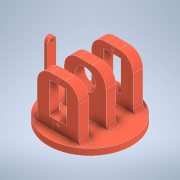
# Autodesk Inventor part: PIEZA 2
Saved by Autodesk Inventor 2021 (Build 250183000, 183)
## iProperties
Created: 2021-03-25
Part Number: PIEZA 2
Material: Generic
Document SubType Name: Modeling
Designer: LRC
Density: 1 g/cm^3
Appearance: Generic
Author: LRC
Autodesk Inventor part; units mm, degrees
ref_plane "YZ Plane" through (0, 0, 0) normal (1, 0, 0) x (0, 1, 0)
ref_plane "XZ Plane" through (0, 0, 0) normal (0, 1, 0) x (-1, 0, 0)
ref_plane "XY Plane" through (0, 0, 0) normal (0, 0, 1) x (1, 0, 0)
sketch "Sketch2" plane through (0, 0, 0) normal (0, 1, 0) x (-1, 0, 0)
  circle A0 centre (0, 0) radius 30
  dimension "d3" = 60
  constraints: 1 centre point, 1 coincident
  measures "d3" diameter of A0
extrude "Extrusion2" add sketch "Sketch2" along normal blind 4.5
sketch "Sketch3" plane through (0, 4.5, 0) normal (0, 1, 0) x (1, 0, 0)
  line L0 (-15, 0) -> (15, 0)
  line L1 (0, -3.5) -> (0, 3.5)
  line L2 (-15, 0) -> (-15, -3.5)
  line L3 (-15, -3.5) -> (15, -3.5)
  line L4 (15, -3.5) -> (15, 3.5)
  line L5 (15, 3.5) -> (-15, 3.5)
  line L6 (-15, 3.5) -> (-15, 0)
  line L7 (-15, -16) -> (-15, -23)
  line L8 (-15, -23) -> (15, -23)
  line L9 (15, -23) -> (15, -16)
  line L10 (15, -16) -> (-15, -16)
  line L11 (-15, 16) -> (-15, 23)
  line L12 (-15, 23) -> (15, 23)
  line L13 (15, 23) -> (15, 16)
  line L14 (15, 16) -> (-15, 16)
  point P0 (0, 0)
  point P1 (0, 0)
  point P2 (0, 0)
  dimension "d6" = 30
  dimension "d7" = 7
  dimension "d8" = 12.5
  dimension "d9" = 7
  dimension "d10" = 30
  dimension "d11" = 7
  constraints: 30 end point, 6 perpendicular, 4 symmetric about line, 3 coincident, 2 midpoint, 2 vertical, 1 horizontal, 1 point on line
  measures "d6" distance of L0.start L0.end
  measures "d7" distance of L1.start L1.end
  measures "d8" distance of L2.end L7.start
  measures "d9" distance of L7.start L7.end
  measures "d10" distance of L7.end L8.end
  measures "d11" distance of L8.end L9.end
extrude "Extrusion3" add sketch "Sketch3" along normal blind 35
fillet "Fillet1" radius 3 6 edges at (15, 4.5, 19.5) (15, 4.5, 0) (15, 4.5, -19.5) (-15, 4.5, 19.5) (-15, 4.5, 0) (-15, 4.5, -19.5)
fillet "Fillet2" radius 10 6 edges at (-15, 39.5, -19.5) (-15, 39.5, 0) (-15, 39.5, 19.5) (15, 39.5, -19.5) (15, 39.5, 0) (15, 39.5, 19.5)
sketch "Sketch4" plane through (0, 4.5, 0) normal (0, 1, 0) x (1, 0, 0)
  line L0 (0, 0) -> (0, 12.5)
  circle A0 centre (0, 12.5) radius 1.5
  line L1 (0, 0) -> (-7, 0)
  circle A1 centre (0, -12.5) radius 1.5
  dimension "d16" = 12.5
  dimension "d17" = 3
  constraints: 4 end point, 2 centre point, 1 coincident, 1 horizontal, 1 symmetric about line, 1 vertical, 1 other
  measures "d16" distance of L0.start L0.end
  measures "d17" diameter of A0
extrude "Extrusion4" cut sketch "Sketch4" against normal up to next
sketch "Sketch5" plane through (-18, 4.5, 23) normal (0, 0, 1) x (1, 0, 0)
  arc A0 (33, 25) -> (23, 35) centre (23, 25) ccw projected
  line L0 (13, 35) -> (23, 35) projected
  arc A1 (13, 35) -> (3, 25) centre (13, 25) ccw projected
  line L1 (3, 3) -> (3, 25) projected
  arc A2 (0, 0) -> (3, 3) centre (0, 3) ccw projected
  line L2 (36, 0) -> (0, 0) projected
  arc A3 (33, 3) -> (36, 0) centre (36, 3) ccw projected
  line L3 (33, 3) -> (33, 25) projected
  line L4 (3, 0) -> (18, 0)
  line L5 (18, 0) -> (18, 5)
  circle A4 centre (18, 5) radius 1
  line L6 (3, 35) -> (18, 35)
  line L7 (13, 35) -> (23, 35) projected
  line L8 (18, 30) -> (18, 35)
  line L9 (18, 35) -> (18, 32.5)
  circle A5 centre (18, 32.5) radius 1
  point P0 (18, -4.5)
  dimension "d20" = 15
  dimension "d21" = 5
  dimension "d22" = 2
  dimension "d23" = 15
  dimension "d24" = 5
  dimension "d25" = 2.5
  dimension "d26" = 2
  constraints: 10 end point, 3 midpoint, 2 centre point, 2 coincident, 1 perpendicular, 1 point on line
  measures "d20" distance of L4.start L4.end
  measures "d21" distance of L4.end L5.end
  measures "d22" diameter of A4
  measures "d23" distance of L6.start L6.end
  measures "d24" distance of L6.end L8.start
  measures "d25" distance of L6.end L9.end
  measures "d26" diameter of A5
extrude "Extrusion5" cut sketch "Sketch5" against normal blind 46 contours A4 | A5 L8 | L8 A5
sketch "Sketch6" plane through (-18, 4.5, 3.5) normal (0, 0, 1) x (1, 0, 0)
  circle A0 centre (18, 32.5) radius 1 projected
  circle A1 centre (18, 32.5) radius 1
  circle A2 centre (18, 5) radius 1
  point P0 (18, -4.5)
  constraints: 2 centre point, 1 coincident
extrude "Extrusion6" add sketch "Sketch6" against normal blind 7
sketch "Sketch7" plane through (-18, 4.5, 23) normal (0, 0, 1) x (1, 0, 0)
  circle A0 centre (18, 5) radius 1 projected
  circle A1 centre (18, 32.5) radius 1 projected
  arc A2 (33, 25) -> (23, 35) centre (23, 25) ccw projected
  line L0 (13, 35) -> (23, 35) projected
  arc A3 (13, 35) -> (3, 25) centre (13, 25) ccw projected
  line L1 (3, 3) -> (3, 25) projected
  arc A4 (0, 0) -> (3, 3) centre (0, 3) ccw projected
  line L2 (36, 0) -> (0, 0) projected
  arc A5 (33, 3) -> (36, 0) centre (36, 3) ccw projected
  line L3 (33, 3) -> (33, 25) projected
  line L4 (23, 35) -> (13, 35) projected
  line L5 (18, 35) -> (18, 30)
  line L6 (11.75, 30) -> (24.25, 30)
  line L7 (11.75, 30) -> (11.75, 7.5)
  line L8 (11.75, 7.5) -> (24.25, 7.5)
  line L9 (24.25, 7.5) -> (24.25, 30)
  point P0 (18, -4.5)
  dimension "d31" = 12.5
  dimension "d32" = 22.5
  constraints: 10 end point, 2 coincident, 2 midpoint, 2 perpendicular, 1 horizontal, 1 vertical
  measures "d31" distance of L6.start L6.end
  measures "d32" distance of L6.start L7.end
extrude "Extrusion7" cut sketch "Sketch7" against normal through all contours L6 L9 L8 L7
sketch "Sketch8" plane through (-18, 4.5, 3.5) normal (0, 0, 1) x (1, 0, 0)
  line L0 (13, 35) -> (23, 35) projected
  line L1 (18, 35) -> (18, 23.75)
  circle A0 centre (18, 23.75) radius 7.5
  line L2 (11.75, 7.5) -> (11.75, 30) projected
  line L3 (11.75, 30) -> (24.25, 30) projected
  line L4 (24.25, 30) -> (24.25, 7.5) projected
  line L5 (24.25, 7.5) -> (11.75, 7.5) projected
  arc A1 (33, 25) -> (23, 35) centre (23, 25) ccw projected
  line L6 (13, 35) -> (23, 35) projected
  arc A2 (13, 35) -> (3, 25) centre (13, 25) ccw projected
  line L7 (3, 3) -> (3, 25) projected
  arc A3 (0, 0) -> (3, 3) centre (0, 3) ccw projected
  line L8 (36, 0) -> (0, 0) projected
  arc A4 (33, 3) -> (36, 0) centre (36, 3) ccw projected
  line L9 (33, 3) -> (33, 25) projected
  line L10 (11.75, 30) -> (11.75, 7.5) projected
  line L11 (11.75, 27.8958) -> (11.75, 30)
  line L12 (11.75, 30) -> (13.8542, 30)
  line L13 (24.25, 30) -> (11.75, 30) projected
  line L14 (24.25, 7.5) -> (24.25, 30) projected
  line L15 (24.25, 27.8958) -> (24.25, 30)
  line L16 (24.25, 30) -> (22.1458, 30)
  line L17 (11.75, 19.6042) -> (11.75, 7.5)
  line L18 (24.25, 7.5) -> (11.75, 7.5) projected
  line L19 (11.75, 7.5) -> (24.25, 7.5)
  line L20 (24.25, 7.5) -> (24.25, 19.6042)
  point P0 (18, -4.5)
  dimension "d35" = 11.25
  dimension "d36" = 15
  constraints: 16 end point, 6 point on circle, 6 point on line, 4 collinear, 1 centre point, 1 coincident, 1 midpoint, 1 vertical
  measures "d35" distance of L1.start L1.end
  measures "d36" diameter of A0
extrude "Extrusion8" add sketch "Sketch8" against normal blind 7 contours L4 L5 L2 A0
extrude "Extrusion9" cut sketch "Sketch8" against normal blind 10 contours A0 L3 L1 | L1 L3 A0 | A0 L4 | L2 A0
extrude "Extrusion10" add sketch "Sketch8" against normal blind 7 contours L3 L4 A0 | A0 L2 L3
sketch "Sketch9" plane through (0, 4.5, 0) normal (0, 1, 0) x (1, 0, 0)
  circle A0 centre (0, 12.5) radius 1.5 projected
  circle A1 centre (0, -12.5) radius 1.5 projected
  line L0 (-18, 23) -> (18, 23) projected
  line L1 (18, 16) -> (18, 23) projected
  line L2 (18, 16) -> (-18, 16) projected
  line L3 (-18, 23) -> (-18, 16) projected
  line L4 (-18, 3.5) -> (18, 3.5) projected
  line L5 (18, -3.5) -> (18, 3.5) projected
  line L6 (18, -3.5) -> (-18, -3.5) projected
  line L7 (-18, 3.5) -> (-18, -3.5) projected
  line L8 (-18, -16) -> (18, -16) projected
  line L9 (18, -23) -> (18, -16) projected
  line L10 (18, -23) -> (-18, -23) projected
  line L11 (-18, -16) -> (-18, -23) projected
  circle A2 centre (0, 0) radius 30 projected
  circle A3 centre (0, 0) radius 30 projected
  line L12 (-30, 0) -> (-28.5642, 0)
  line L13 (-30, 0) -> (-27.3496, 0)
  line L14 (-27.3496, 0) -> (-27.3496, 3)
  line L15 (-27.3496, 3) -> (-29.8496, 3)
  line L16 (-27.3496, 0) -> (-27.3496, -3)
  line L17 (-27.3496, -3) -> (-29.8496, -3)
  dimension "d45" = 2.5
  dimension "d46" = 6
  constraints: 12 end point, 4 horizontal, 2 coincident, 2 point on circle, 2 symmetric about line, 1 vertical
  measures "d45" distance of L14.end L15.end
  measures "d46" distance between parallel lines of L15 L17
extrude "Extrusion11" add sketch "Sketch9" along normal blind 35 contours L15 L14 L13 L12 A2 | A2 L12 L13 L16 L17
fillet "Fillet3" radius 3 2 edges at (-28.5996, 39.5, -3) (-28.5996, 39.5, 3)
sketch "Sketch10" plane through (-27.3496, 4.5, 3) normal (1, 0, 0) x (0, 0, -1)
  line L0 (6, 0) -> (6, 32) projected
  line L1 (0, 0) -> (6, 0) projected
  line L2 (0, 0) -> (0, 32) projected
  line L3 (33, -4.5) -> (-27, -4.5) projected
  circle A0 centre (3, 32) radius 3
  circle A1 centre (3, 32) radius 1.5
  point P0 (3, -4.5)
  dimension "d51" = 6
  dimension "d52" = 3
  constraints: 2 centre point, 1 coincident, 2 other
  measures "d51" diameter of A0
  measures "d52" diameter of A1
extrude "Extrusion12" cut sketch "Sketch10" against normal blind 10 contours A1
body "Solid2"
